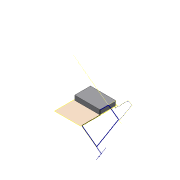
# Autodesk Inventor part: PTFEFilter_clamp
Saved by Autodesk Inventor 2014 (Build 180170000, 170)
## iProperties
Created: 2016-08-28
Part Number: PTFEFilter_clamp
Material: Generic
Document SubType Name: Modeling
Designer: Camilo
Density: 1 g/cm^3
Appearance: Default
d0: 5.000 mm
d1: 0.120 mm
d2: 1.500 mm
d3: 0.00 deg
d4: 0.120 mm
d5: 1.000 mm
d6: 1.000 mm
d7: 0.00 deg
Author: Camilo
Autodesk Inventor part; units mm, degrees
ref_plane "YZ Plane" through (0, 0, 0) normal (1, 0, 0) x (0, 1, 0)
ref_plane "XZ Plane" through (0, 0, 0) normal (0, 1, 0) x (-1, 0, 0)
ref_plane "XY Plane" through (0, 0, 0) normal (0, 0, 1) x (1, 0, 0)
ref_plane "Work Plane1" through (0, 0, 0) normal (0, 0, 1) x (1, 0, 0)
sketch "Sketch1" plane through (0, 0, 0) normal (0, 0, 1) x (1, 0, 0)
  line L0 (4, -5.5111) -> (4, 5.5111) construction
  line L1 (4, 5.5111) -> (-4, 5.5111) construction
  line L2 (-4, 5.5111) -> (-4, -5.5111) construction
  line L3 (-4, -5.5111) -> (4, -5.5111) construction
  line L4 (-4, 5.5111) -> (4.1522, 5.5111) construction
  line L5 (4.1522, 5.5111) -> (4.1522, 0.5111) construction
  line L6 (4.1522, 0.5111) -> (-4, 0.5111) construction
  line L7 (-4, 0.5111) -> (-4, 5.5111) construction
  line L8 (-4.12, 0.3911) -> (4.2722, 0.3911)
  line L9 (4.2722, 0.3911) -> (4.2722, 5.6311)
  line L10 (4.2722, 5.6311) -> (-4.12, 5.6311)
  line L11 (-4.12, 5.6311) -> (-4.12, 0.3911)
  point P0 (0, 0)
  dimension "d0" = 5
  dimension "d1" = 0.12
  constraints: 16 end point, 3 other
  measures "d0" distance of L4.end L5.end
  measures "d1" distance between parallel lines of L5 L9
extrude "Extrusion1" add sketch "Sketch1" along normal blind 1.5
sketch "Sketch2" plane through (4.2722, 0.3911, 0) normal (1, 0, 0) x (0, 0, -1)
  line L0 (-1.5, 0) -> (-1.5, 5.24) construction
  line L1 (4.4205, 6.1762) -> (4.9103, 6.459) construction
  line L2 (4.9103, 6.459) -> (2.5, 10.6336) construction
  line L3 (2.5, 10.6336) -> (0.5, 9.4789) construction
  line L4 (0.5, 9.4789) -> (0.5, 5.12) construction
  line L5 (0.5, 5.12) -> (0, 5.12) construction
  line L6 (0, -5.9023) -> (0, 5.12) construction
  line L7 (0.5, -5.9023) -> (0, -5.9023) construction
  line L8 (8.6705, -1.185) -> (0.5, -5.9023) construction
  line L9 (8.6705, -1.185) -> (4.4205, 6.1762) construction
  line L10 (0.4678, -5.7823) -> (0.12, -5.7823) construction
  line L11 (0.12, -5.7823) -> (0.12, 5) construction
  line L12 (0.12, 5) -> (0.62, 5) construction
  line L13 (0.62, 5) -> (0.62, 9.4097) construction
  line L14 (0.62, 9.4097) -> (2.4561, 10.4697) construction
  line L15 (2.4561, 10.4697) -> (4.7463, 6.5029) construction
  line L16 (4.7463, 6.5029) -> (4.2566, 6.2201) construction
  line L17 (4.2566, 6.2201) -> (8.5066, -1.1411) construction
  line L18 (8.5066, -1.1411) -> (0.4678, -5.7823) construction
  line L19 (6.2093, 7.209) -> (-21.3823, -8.721) construction
  line L20 (4.3166, 6.1162) -> (-1.5, 2.758)
  line L21 (-1.5, 2.758) -> (-1.5, 0)
  line L22 (-1.5, 0) -> (0.12, 0)
  line L23 (8.5066, -1.1411) -> (0, -6.0524)
  line L24 (0, -6.0524) -> (0, 0)
  line L25 (8.5066, -1.1411) -> (4.3166, 6.1162)
  line L26 (3.4506, 5.6162) -> (7.6406, -1.6411)
  line L27 (0, -6.0524) -> (0, 0)
  line L28 (0, 0) -> (-1.5, 0)
  point P0 (0, -0.3911)
  dimension "d4" = 0.12
  dimension "d5" = 1
  constraints: 36 end point, 8 point on line, 8 other
  measures "d4" distance between parallel lines of L18 L8
  measures "d5" distance between parallel lines of L17 L26
extrude "Extrusion2" add sketch "Sketch2" along normal blind 1 contours L26 L23 L24 L22 L21 L20
ref_plane "Work Plane2" through (0.0761, 5.6311, 1.5) normal (1, 0, 0) x (0, 0, -1)
mirror "Mirror1" about plane through (0.0761, 5.6311, 1.5) normal (1, 0, 0) of "Extrusion2"
body "Solid1"
